Autodesk Fusion 360 part; units mm, degrees
(part 7 of 8)
  spline S13 degree 5 poles (6.6784, -162.4797) (6.7115, -162.4181) (6.7775, -162.295) (6.8761, -162.1103) (7.0066, -161.8637) (7.1683, -161.555) (7.3285, -161.246) (7.4872, -160.9366) (7.6444, -160.6268) (7.8, -160.3167) (7.9541, -160.0061) (8.1066, -159.6952) (8.2576, -159.3839) (8.407, -159.0722) (8.5549, -158.7602) (8.7011, -158.4478) (8.8457, -158.1351) (8.9887, -157.822) (9.1301, -157.5085) (9.2698, -157.1947) (9.4079, -156.8806) (9.5443, -156.5661) (9.679, -156.2513) (9.812, -155.9362) (9.9433, -155.6207) (10.0728, -155.3049) (10.2006, -154.9888) (10.3267, -154.6723) (10.4509, -154.3556) (10.5734, -154.0385) (10.694, -153.7211) (10.8129, -153.4035) (10.9298, -153.0855) (11.0449, -152.7672) (11.158, -152.4487) (11.2693, -152.1299) (11.3786, -151.8107) (11.486, -151.4913) (11.5914, -151.1717) (11.6948, -150.8517) (11.7962, -150.5315) (11.8955, -150.2111) (11.9926, -149.8904) (12.0876, -149.5694) (12.1804, -149.2482) (12.271, -148.9268) (12.3594, -148.6051) (12.4457, -148.2833) (12.5297, -147.9611) (12.6115, -147.6388) (12.6907, -147.3163) (12.7674, -146.9936) (12.8414, -146.6706) (12.9127, -146.3475) (12.9813, -146.0243) (13.0473, -145.7008) (13.1109, -145.3772) (13.1722, -145.0534) (13.231, -144.7295) (13.2868, -144.4055) (13.3392, -144.0813) (13.3875, -143.757) (13.4313, -143.4326) (13.4707, -143.1082) (13.5063, -142.7837) (13.539, -142.4591) (13.5696, -142.1346) (13.598, -141.81) (13.6235, -141.4854) (13.6434, -141.161) (13.6541, -140.8368) (13.6525, -140.5776) (13.6443, -140.3834) (13.6355, -140.254) (13.6303, -140.1893) knots -1 -1 -1 -1 -1 -1 -0.98571429 -0.97142857 -0.95714286 -0.94285714 -0.92857143 -0.91428571 -0.9 -0.88571429 -0.87142857 -0.85714286 -0.84285714 -0.82857143 -0.81428571 -0.8 -0.78571429 -0.77142857 -0.75714286 -0.74285714 -0.72857143 -0.71428571 -0.7 -0.68571429 -0.67142857 -0.65714286 -0.64285714 -0.62857143 -0.61428571 -0.6 -0.58571429 -0.57142857 -0.55714286 -0.54285714 -0.52857143 -0.51428571 -0.5 -0.48571429 -0.47142857 -0.45714286 -0.44285714 -0.42857143 -0.41428571 -0.4 -0.38571429 -0.37142857 -0.35714286 -0.34285714 -0.32857143 -0.31428571 -0.3 -0.28571429 -0.27142857 -0.25714286 -0.24285714 -0.22857143 -0.21428571 -0.2 -0.18571429 -0.17142857 -0.15714286 -0.14285714 -0.12857143 -0.11428571 -0.1 -0.08571429 -0.07142857 -0.05714286 -0.04285714 -0.02857143 -0.01428571 0 0 0 0 0 0
  line L13 (13.6303, -140.1893) -> (13.2679, -135.6821)
  arc A27 (14.7048, -133.974) -> (13.2679, -135.6821) centre (14.8503, -135.5548) ccw
  arc A28 (14.7048, -133.974) -> (25.331, -132.5751) centre (2.1352, 2.5578) ccw
  arc A29 (27.1609, -133.853) -> (25.331, -132.5751) centre (25.5995, -134.1397) ccw
  line L14 (27.1609, -133.853) -> (27.9775, -138.3004)
  spline S14 degree 5 poles (27.9775, -138.3004) (27.9892, -138.3643) (28.0142, -138.4915) (28.0566, -138.6813) (28.1221, -138.9321) (28.2164, -139.2425) (28.3195, -139.5507) (28.4281, -139.8576) (28.5397, -140.1637) (28.6532, -140.4693) (28.7687, -140.7744) (28.8871, -141.0786) (29.0091, -141.3818) (29.1355, -141.6837) (29.266, -141.9845) (29.4005, -142.284) (29.5383, -142.5826) (29.6789, -142.8803) (29.8219, -143.1771) (29.9671, -143.4733) (30.1146, -143.7686) (30.2646, -144.0631) (30.417, -144.3568) (30.5721, -144.6495) (30.7297, -144.9414) (30.8897, -145.2324) (31.0521, -145.5226) (31.2166, -145.812) (31.3832, -146.1006) (31.5519, -146.3884) (31.7227, -146.6754) (31.8954, -146.9617) (32.0702, -147.2471) (32.2471, -147.5317) (32.4259, -147.8156) (32.6067, -148.0986) (32.7893, -148.3809) (32.9739, -148.6624) (33.1603, -148.9431) (33.3485, -149.2231) (33.5385, -149.5023) (33.7302, -149.7807) (33.9238, -150.0583) (34.119, -150.3352) (34.316, -150.6113) (34.5147, -150.8866) (34.7151, -151.1611) (34.9171, -151.4349) (35.1207, -151.708) (35.326, -151.9803) (35.5329, -152.2518) (35.7413, -152.5225) (35.9514, -152.7925) (36.1629, -153.0617) (36.3761, -153.3302) (36.5907, -153.5979) (36.8069, -153.8648) (37.0246, -154.131) (37.2438, -154.3964) (37.4644, -154.6611) (37.6865, -154.925) (37.91, -155.1881) (38.135, -155.4505) (38.3614, -155.7121) (38.5893, -155.9729) (38.8185, -156.233) (39.0491, -156.4923) (39.2811, -156.7509) (39.5144, -157.0087) (39.7491, -157.2657) (39.9852, -157.522) (40.1751, -157.7264) (40.3182, -157.8793) (40.4138, -157.9811) (40.4617, -158.032) knots 0 0 0 0 0 0 0.01428571 0.02857143 0.04285714 0.05714286 0.07142857 0.08571429 0.1 0.11428571 0.12857143 0.14285714 0.15714286 0.17142857 0.18571429 0.2 0.21428571 0.22857143 0.24285714 0.25714286 0.27142857 0.28571429 0.3 0.31428571 0.32857143 0.34285714 0.35714286 0.37142857 0.38571429 0.4 0.41428571 0.42857143 0.44285714 0.45714286 0.47142857 0.48571429 0.5 0.51428571 0.52857143 0.54285714 0.55714286 0.57142857 0.58571429 0.6 0.61428571 0.62857143 0.64285714 0.65714286 0.67142857 0.68571429 0.7 0.71428571 0.72857143 0.74285714 0.75714286 0.77142857 0.78571429 0.8 0.81428571 0.82857143 0.84285714 0.85714286 0.87142857 0.88571429 0.9 0.91428571 0.92857143 0.94285714 0.95714286 0.97142857 0.98571429 1 1 1 1 1 1
  arc A30 (40.4617, -158.032) -> (49.2384, -155.6803) centre (2.1352, 2.5578) ccw
  spline S15 degree 5 poles (49.2384, -155.6803) (49.2545, -155.6123) (49.2864, -155.4763) (49.3338, -155.2723) (49.3961, -155.0003) (49.4724, -154.6604) (49.5471, -154.3204) (49.6203, -153.9805) (49.6919, -153.6406) (49.762, -153.3007) (49.8305, -152.9608) (49.8973, -152.621) (49.9626, -152.2813) (50.0263, -151.9416) (50.0883, -151.6019) (50.1487, -151.2623) (50.2074, -150.9228) (50.2645, -150.5834) (50.32, -150.244) (50.3737, -149.9047) (50.4258, -149.5656) (50.4761, -149.2265) (50.5247, -148.8876) (50.5716, -148.5487) (50.6168, -148.21) (50.6602, -147.8715) (50.7018, -147.533) (50.7417, -147.1948) (50.7797, -146.8566) (50.816, -146.5187) (50.8504, -146.1809) (50.8829, -145.8433) (50.9136, -145.5059) (50.9424, -145.1687) (50.9692, -144.8317) (50.9942, -144.4949) (51.0172, -144.1584) (51.0383, -143.8221) (51.0573, -143.486) (51.0744, -143.1502) (51.0894, -142.8147) (51.1024, -142.4795) (51.1132, -142.1446) (51.1219, -141.81) (51.1284, -141.4757) (51.1327, -141.1418) (51.1349, -140.8082) (51.1349, -140.4749) (51.1327, -140.142) (51.1282, -139.8095) (51.1213, -139.4775) (51.1119, -139.1459) (51.0998, -138.8148) (51.085, -138.4843) (51.0675, -138.1543) (51.0476, -137.8248) (51.0253, -137.4957) (51.0007, -137.1671) (50.9736, -136.839) (50.9437, -136.5116) (50.9104, -136.1849) (50.8731, -135.8592) (50.8315, -135.5345) (50.7856, -135.2109) (50.736, -134.8882) (50.6836, -134.5663) (50.6291, -134.2449) (50.5726, -133.924) (50.5132, -133.6039) (50.4484, -133.2854) (50.3749, -132.9694) (50.3062, -132.7195) (50.248, -132.534) (50.2061, -132.4113) (50.1843, -132.3501) knots -1 -1 -1 -1 -1 -1 -0.98571429 -0.97142857 -0.95714286 -0.94285714 -0.92857143 -0.91428571 -0.9 -0.88571429 -0.87142857 -0.85714286 -0.84285714 -0.82857143 -0.81428571 -0.8 -0.78571429 -0.77142857 -0.75714286 -0.74285714 -0.72857143 -0.71428571 -0.7 -0.68571429 -0.67142857 -0.65714286 -0.64285714 -0.62857143 -0.61428571 -0.6 -0.58571429 -0.57142857 -0.55714286 -0.54285714 -0.52857143 -0.51428571 -0.5 -0.48571429 -0.47142857 -0.45714286 -0.44285714 -0.42857143 -0.41428571 -0.4 -0.38571429 -0.37142857 -0.35714286 -0.34285714 -0.32857143 -0.31428571 -0.3 -0.28571429 -0.27142857 -0.25714286 -0.24285714 -0.22857143 -0.21428571 -0.2 -0.18571429 -0.17142857 -0.15714286 -0.14285714 -0.12857143 -0.11428571 -0.1 -0.08571429 -0.07142857 -0.05714286 -0.04285714 -0.02857143 -0.01428571 0 0 0 0 0 0
  line L15 (50.1843, -132.3501) -> (48.6677, -128.0903)
  arc A31 (49.6135, -126.0686) -> (48.6677, -128.0903) centre (50.1633, -127.5578) ccw
  arc A32 (49.6135, -126.0686) -> (59.5156, -121.967) centre (2.1352, 2.5578) ccw
  arc A33 (61.6139, -122.7278) -> (59.5156, -121.967) centre (60.1799, -123.4088) ccw
  line L16 (61.6139, -122.7278) -> (63.5537, -126.8123)
  spline S16 degree 5 poles (63.5537, -126.8123) (63.5816, -126.871) (63.6387, -126.9874) (63.7287, -127.1598) (63.8569, -127.385) (64.0283, -127.6604) (64.2077, -127.9315) (64.392, -128.1998) (64.579, -128.4666) (64.7677, -128.7325) (64.9583, -128.9972) (65.1514, -129.2604) (65.3477, -129.5217) (65.5479, -129.7807) (65.7519, -130.0373) (65.9593, -130.2919) (66.1697, -130.5446) (66.3825, -130.7957) (66.5975, -131.0455) (66.8144, -131.294) (67.0333, -131.5411) (67.2544, -131.7867) (67.4776, -132.0309) (67.7032, -132.2736) (67.9309, -132.5147) (68.1608, -132.7544) (68.3928, -132.9927) (68.6266, -133.2296) (68.8623, -133.4652) (69.0997, -133.6996) (69.3389, -133.9326) (69.5799, -134.1644) (69.8226, -134.3949) (70.0671, -134.6241) (70.3133, -134.8519) (70.5611, -135.0786) (70.8107, -135.3039) (71.0618, -135.5281) (71.3145, -135.751) (71.5687, -135.9727) (71.8245, -136.1932) (72.0818, -136.4125) (72.3406, -136.6305) (72.6008, -136.8474) (72.8626, -137.0631) (73.1257, -137.2777) (73.3903, -137.491) (73.6563, -137.7032) (73.9237, -137.9142) (74.1924, -138.1241) (74.4625, -138.3328) (74.734, -138.5404) (75.0067, -138.7468) (75.2808, -138.9521) (75.5561, -139.1562) (75.8328, -139.3593) (76.1107, -139.5611) (76.3898, -139.7619) (76.6702, -139.9616) (76.9518, -140.1601) (77.2347, -140.3575) (77.5187, -140.5538) (77.8039, -140.749) (78.0903, -140.9431) (78.3779, -141.1361) (78.6666, -141.328) (78.9565, -141.5188) (79.2475, -141.7085) (79.5396, -141.8971) (79.8328, -142.0846) (80.1272, -142.2711) (80.3635, -142.4194) (80.5413, -142.5301) (80.66, -142.6037) (80.7195, -142.6404) knots 0 0 0 0 0 0 0.01428571 0.02857143 0.04285714 0.05714286 0.07142857 0.08571429 0.1 0.11428571 0.12857143 0.14285714 0.15714286 0.17142857 0.18571429 0.2 0.21428571 0.22857143 0.24285714 0.25714286 0.27142857 0.28571429 0.3 0.31428571 0.32857143 0.34285714 0.35714286 0.37142857 0.38571429 0.4 0.41428571 0.42857143 0.44285714 0.45714286 0.47142857 0.48571429 0.5 0.51428571 0.52857143 0.54285714 0.55714286 0.57142857 0.58571429 0.6 0.61428571 0.62857143 0.64285714 0.65714286 0.67142857 0.68571429 0.7 0.71428571 0.72857143 0.74285714 0.75714286 0.77142857 0.78571429 0.8 0.81428571 0.82857143 0.84285714 0.85714286 0.87142857 0.88571429 0.9 0.91428571 0.92857143 0.94285714 0.95714286 0.97142857 0.98571429 1 1 1 1 1 1
  arc A34 (80.7195, -142.6404) -> (88.5885, -138.0973) centre (2.1352, 2.5578) ccw
  spline S17 degree 5 poles (88.5885, -138.0973) (88.5864, -138.0274) (88.582, -137.8878) (88.575, -137.6785) (88.5647, -137.3997) (88.5504, -137.0515) (88.5347, -136.7038) (88.5174, -136.3565) (88.4986, -136.0097) (88.4783, -135.6632) (88.4565, -135.3172) (88.4331, -134.9717) (88.4082, -134.6266) (88.3818, -134.282) (88.3538, -133.9379) (88.3243, -133.5942) (88.2931, -133.2511) (88.2604, -132.9084) (88.2261, -132.5663) (88.1902, -132.2247) (88.1527, -131.8836) (88.1136, -131.543) (88.0729, -131.2031) (88.0305, -130.8636) (87.9864, -130.5248) (87.9407, -130.1865) (87.8933, -129.8488) (87.8443, -129.5118) (87.7935, -129.1753) (87.7411, -128.8395) (87.6869, -128.5043) (87.6309, -128.1698) (87.5732, -127.836) (87.5137, -127.5028) (87.4525, -127.1703) (87.3894, -126.8386) (87.3245, -126.5076) (87.2578, -126.1773) (87.1893, -125.8477) (87.1189, -125.519) (87.0465, -125.191) (86.9723, -124.8638) (86.896, -124.5375) (86.8178, -124.2121) (86.7376, -123.8875) (86.6553, -123.5638) (86.5711, -123.241) (86.4849, -122.9191) (86.3966, -122.5982) (86.3062, -122.2782) (86.2136, -121.9592) (86.1187, -121.6414) (86.0213, -121.3247) (85.9214, -121.0093) (85.8192, -120.695) (85.7147, -120.3819) (85.608, -120.0698) (85.4991, -119.7588) (85.3881, -119.4489) (85.2744, -119.1403) (85.1577, -118.8334) (85.0374, -118.5284) (84.9132, -118.2256) (84.7851, -117.9249) (84.6536, -117.6261) (84.5197, -117.3287) (84.3838, -117.0323) (84.2462, -116.737) (84.106, -116.4432) (83.961, -116.1523) (83.8082, -115.8661) (83.6772, -115.6425) (83.5729, -115.4784) (83.5006, -115.3707) (83.4638, -115.3172) knots -1 -1 -1 -1 -1 -1 -0.98571429 -0.97142857 -0.95714286 -0.94285714 -0.92857143 -0.91428571 -0.9 -0.88571429 -0.87142857 -0.85714286 -0.84285714 -0.82857143 -0.81428571 -0.8 -0.78571429 -0.77142857 -0.75714286 -0.74285714 -0.72857143 -0.71428571 -0.7 -0.68571429 -0.67142857 -0.65714286 -0.64285714 -0.62857143 -0.61428571 -0.6 -0.58571429 -0.57142857 -0.55714286 -0.54285714 -0.52857143 -0.51428571 -0.5 -0.48571429 -0.47142857 -0.45714286 -0.44285714 -0.42857143 -0.41428571 -0.4 -0.38571429 -0.37142857 -0.35714286 -0.34285714 -0.32857143 -0.31428571 -0.3 -0.28571429 -0.27142857 -0.25714286 -0.24285714 -0.22857143 -0.21428571 -0.2 -0.18571429 -0.17142857 -0.15714286 -0.14285714 -0.12857143 -0.11428571 -0.1 -0.08571429 -0.07142857 -0.05714286 -0.04285714 -0.02857143 -0.01428571 0 0 0 0 0 0
  line L17 (83.4638, -115.3172) -> (80.8964, -111.5951)
  arc A35 (81.2867, -109.3974) -> (80.8964, -111.5951) centre (82.2032, -110.6937) ccw
  arc A36 (81.2867, -109.3974) -> (89.7898, -102.8728) centre (2.1352, 2.5578) ccw
  arc A37 (92.0135, -103.0646) -> (89.7898, -102.8728) centre (90.8047, -104.0935) ccw
  line L18 (92.0135, -103.0646) -> (94.9444, -106.5079)
  spline S18 degree 5 poles (94.9444, -106.5079) (94.9865, -106.5573) (95.0718, -106.655) (95.2033, -106.7982) (95.3854, -106.9826) (95.6223, -107.2043) (95.8657, -107.4196) (96.1132, -107.6311) (96.3629, -107.8404) (96.614, -108.0484) (96.8666, -108.2547) (97.1212, -108.459) (97.3785, -108.6606) (97.6389, -108.8589) (97.9023, -109.0541) (98.1686, -109.2463) (98.4372, -109.4359) (98.7078, -109.6234) (98.9801, -109.809) (99.2539, -109.9929) (99.5293, -110.1749) (99.8064, -110.355) (100.0853, -110.5331) (100.3659, -110.7091) (100.6483, -110.8831) (100.9325, -111.0551) (101.2182, -111.2252) (101.5053, -111.3935) (101.794, -111.5601) (102.084, -111.725) (102.3753, -111.8883) (102.6681, -112.0498) (102.9622, -112.2096) (103.2576, -112.3676) (103.5544, -112.524) (103.8525, -112.6788) (104.1518, -112.8319) (104.4524, -112.9834) (104.7542, -113.1333) (105.0571, -113.2817) (105.3613, -113.4284) (105.6665, -113.5737) (105.973, -113.7173) (106.2805, -113.8595) (106.5891, -114.0001) (106.8989, -114.1392) (107.2097, -114.2768) (107.5215, -114.4129) (107.8344, -114.5475) (108.1483, -114.6807) (108.4632, -114.8124) (108.7791, -114.9426) (109.096, -115.0714) (109.4139, -115.1988) (109.7327, -115.3247) (110.0524, -115.4492) (110.3731, -115.5723) (110.6947, -115.694) (111.0172, -115.8143) (111.3406, -115.9331) (111.6649, -116.0506) (111.9901, -116.1667) (112.3161, -116.2815) (112.643, -116.3948) (112.9707, -116.5068) (113.2993, -116.6174) (113.6286, -116.7267) (113.9588, -116.8346) (114.2898, -116.9412) (114.6216, -117.0464) (114.9542, -117.1504) (115.2208, -117.2324) (115.4212, -117.2933) (115.5549, -117.3337) (115.6218, -117.3538) knots 0 0 0 0 0 0 0.01428571 0.02857143 0.04285714 0.05714286 0.07142857 0.08571429 0.1 0.11428571 0.12857143 0.14285714 0.15714286 0.17142857 0.18571429 0.2 0.21428571 0.22857143 0.24285714 0.25714286 0.27142857 0.28571429 0.3 0.31428571 0.32857143 0.34285714 0.35714286 0.37142857 0.38571429 0.4 0.41428571 0.42857143 0.44285714 0.45714286 0.47142857 0.48571429 0.5 0.51428571 0.52857143 0.54285714 0.55714286 0.57142857 0.58571429 0.6 0.61428571 0.62857143 0.64285714 0.65714286 0.67142857 0.68571429 0.7 0.71428571 0.72857143 0.74285714 0.75714286 0.77142857 0.78571429 0.8 0.81428571 0.82857143 0.84285714 0.85714286 0.87142857 0.88571429 0.9 0.91428571 0.92857143 0.94285714 0.95714286 0.97142857 0.98571429 1 1 1 1 1 1
  arc A38 (115.6218, -117.3538) -> (122.0469, -110.9288) centre (2.1352, 2.5578) ccw
  spline S19 degree 5 poles (122.0469, -110.9288) (122.0267, -110.8619) (121.9864, -110.7282) (121.9254, -110.5278) (121.8434, -110.2611) (121.7395, -109.9286) (121.6342, -109.5968) (121.5277, -109.2658) (121.4197, -108.9356) (121.3105, -108.6062) (121.1998, -108.2777) (121.0878, -107.95) (120.9745, -107.6231) (120.8598, -107.297) (120.7437, -106.9719) (120.6262, -106.6476) (120.5073, -106.3242) (120.387, -106.0017) (120.2653, -105.6801) (120.1423, -105.3594) (120.0177, -105.0396) (119.8918, -104.7208) (119.7645, -104.403) (119.6357, -104.0861) (119.5054, -103.7702) (119.3737, -103.4553) (119.2406, -103.1414) (119.1059, -102.8285) (118.9698, -102.5166) (118.8322, -102.2058) (118.6931, -101.8961) (118.5525, -101.5875) (118.4104, -101.2799) (118.2667, -100.9735) (118.1215, -100.6682) (117.9747, -100.3641) (117.8263, -100.0612) (117.6764, -99.7594) (117.5249, -99.4588) (117.3718, -99.1595) (117.2171, -98.8614) (117.0607, -98.5646) (116.9026, -98.2691) (116.7428, -97.975) (116.5813, -97.6823) (116.4181, -97.3909) (116.2532, -97.1009) (116.0866, -96.8123) (115.9182, -96.5251) (115.7481, -96.2394) (115.5761, -95.9553) (115.4021, -95.6729) (115.2261, -95.3922) (115.048, -95.1134) (114.8679, -94.8363) (114.6859, -94.5609) (114.5021, -94.287) (114.3164, -94.0148) (114.1289, -93.7442) (113.9393, -93.4756) (113.7471, -93.2093) (113.552, -92.9459) (113.3536, -92.6855) (113.1521, -92.4282) (112.9478, -92.1736) (112.7414, -91.921) (112.5335, -91.6699) (112.3241, -91.4202) (112.1126, -91.1727) (111.8973, -90.9293) (111.6756, -90.6924) (111.4912, -90.5103) (111.348, -90.3788) (111.2503, -90.2934) (111.2009, -90.2514) knots -1 -1 -1 -1 -1 -1 -0.98571429 -0.97142857 -0.95714286 -0.94285714 -0.92857143 -0.91428571 -0.9 -0.88571429 -0.87142857 -0.85714286 -0.84285714 -0.82857143 -0.81428571 -0.8 -0.78571429 -0.77142857 -0.75714286 -0.74285714 -0.72857143 -0.71428571 -0.7 -0.68571429 -0.67142857 -0.65714286 -0.64285714 -0.62857143 -0.61428571 -0.6 -0.58571429 -0.57142857 -0.55714286 -0.54285714 -0.52857143 -0.51428571 -0.5 -0.48571429 -0.47142857 -0.45714286 -0.44285714 -0.42857143 -0.41428571 -0.4 -0.38571429 -0.37142857 -0.35714286 -0.34285714 -0.32857143 -0.31428571 -0.3 -0.28571429 -0.27142857 -0.25714286 -0.24285714 -0.22857143 -0.21428571 -0.2 -0.18571429 -0.17142857 -0.15714286 -0.14285714 -0.12857143 -0.11428571 -0.1 -0.08571429 -0.07142857 -0.05714286 -0.04285714 -0.02857143 -0.01428571 0 0 0 0 0 0
  line L19 (111.2009, -90.2514) -> (107.7576, -87.3205)
  arc A39 (107.5658, -85.0967) -> (107.7576, -87.3205) centre (108.7866, -86.1116) ccw
  arc A40 (107.5658, -85.0967) -> (114.0905, -76.5937) centre (2.1352, 2.5578) ccw
  arc A41 (116.2881, -76.2033) -> (114.0905, -76.5937) centre (115.3867, -77.5101) ccw
  line L20 (116.2881, -76.2033) -> (120.0103, -78.7708)
  spline S20 degree 5 poles (120.0103, -78.7708) (120.0637, -78.8076) (120.1714, -78.8799) (120.3355, -78.9842) (120.5592, -79.1151) (120.8453, -79.268) (121.1362, -79.413) (121.43, -79.5532) (121.7253, -79.6908) (122.0217, -79.8266) (122.3191, -79.9606) (122.6179, -80.092) (122.9186, -80.2201) (123.2215, -80.3443) (123.5264, -80.4646) (123.8333, -80.5814) (124.1419, -80.695) (124.4518, -80.8061) (124.7628, -80.9149) (125.0749, -81.0216) (125.3881, -81.1262) (125.7023, -81.2284) (126.0178, -81.3283) (126.3344, -81.4256) (126.6522, -81.5206) (126.9712, -81.6132) (127.2912, -81.7036) (127.6122, -81.7919) (127.9341, -81.8781) (128.2569, -81.9623) (128.5805, -82.0446) (128.9051, -82.1248) (129.2305, -82.203) (129.5569, -82.2793) (129.884, -82.3535) (130.212, -82.4258) (130.5408, -82.4962) (130.8703, -82.5648) (131.2006, -82.6315) (131.5316, -82.6964) (131.8634, -82.7594) (132.1958, -82.8207) (132.529, -82.8802) (132.8628, -82.9379) (133.1974, -82.9938) (133.5325, -83.048) (133.8684, -83.1005) (134.2048, -83.1513) (134.5419, -83.2003) (134.8795, -83.2477) (135.2178, -83.2934) (135.5567, -83.3374) (135.8961, -83.3798) (136.2361, -83.4206) (136.5766, -83.4597) (136.9177, -83.4972) (137.2593, -83.5331) (137.6014, -83.5674) (137.9441, -83.6001) (138.2872, -83.6312) (138.6309, -83.6608) (138.975, -83.6888) (139.3196, -83.7152) (139.6647, -83.7401) (140.0103, -83.7634) (140.3563, -83.7853) (140.7027, -83.8056) (141.0496, -83.8244) (141.3969, -83.8416) (141.7446, -83.8574) (142.0927, -83.8717) (142.3715, -83.8819) (142.5808, -83.889) (142.7205, -83.8933) (142.7903, -83.8954) knots 0 0 0 0 0 0 0.01428571 0.02857143 0.04285714 0.05714286 0.07142857 0.08571429 0.1 0.11428571 0.12857143 0.14285714 0.15714286 0.17142857 0.18571429 0.2 0.21428571 0.22857143 0.24285714 0.25714286 0.27142857 0.28571429 0.3 0.31428571 0.32857143 0.34285714 0.35714286 0.37142857 0.38571429 0.4 0.41428571 0.42857143 0.44285714 0.45714286 0.47142857 0.48571429 0.5 0.51428571 0.52857143 0.54285714 0.55714286 0.57142857 0.58571429 0.6 0.61428571 0.62857143 0.64285714 0.65714286 0.67142857 0.68571429 0.7 0.71428571 0.72857143 0.74285714 0.75714286 0.77142857 0.78571429 0.8 0.81428571 0.82857143 0.84285714 0.85714286 0.87142857 0.88571429 0.9 0.91428571 0.92857143 0.94285714 0.95714286 0.97142857 0.98571429 1 1 1 1 1 1
  arc A42 (142.7903, -83.8954) -> (147.3335, -76.0264) centre (2.1352, 2.5578) ccw
  spline S21 degree 5 poles (147.3335, -76.0264) (147.2967, -75.967) (147.2231, -75.8483) (147.1124, -75.6705) (146.9641, -75.4342) (146.7777, -75.1398) (146.5902, -74.8466) (146.4015, -74.5545) (146.2118, -74.2635) (146.021, -73.9736) (145.8291, -73.6849) (145.6361, -73.3973) (145.442, -73.1109) (145.2468, -72.8257) (145.0505, -72.5416) (144.8531, -72.2588) (144.6546, -71.9772) (144.4549, -71.6968) (144.2542, -71.4176) (144.0523, -71.1397) (143.8493, -70.8631) (143.6451, -70.5877) (143.4398, -70.3137) (143.2334, -70.0409) (143.0258, -69.7695) (142.8171, -69.4994) (142.6073, -69.2307) (142.3962, -68.9633) (142.1841, -68.6973) (141.9707, -68.4327) (141.7562, -68.1695) (141.5405, -67.9078) (141.3236, -67.6475) (141.1055, -67.3887) (140.8862, -67.1315) (140.6657, -66.8757) (140.444, -66.6214) (140.2211, -66.3687) (139.997, -66.1176) (139.7716, -65.8681) (139.545, -65.6202) (139.3171, -65.374) (139.0879, -65.1296) (138.8574, -64.8868) (138.6257, -64.6459) (138.3926, -64.4067) (138.1583, -64.1692) (137.9227, -63.9336) (137.6857, -63.6998) (137.4474, -63.4678) (137.2078, -63.2379) (136.9666, -63.0101) (136.7239, -62.7846) (136.4798, -62.5613) (136.2341, -62.3403) (135.987, -62.1214) (135.7385, -61.9045) (135.4888, -61.6895) (135.2376, -61.4767) (134.9849, -61.2663) (134.7304, -61.0588) (134.4737, -60.8549) (134.2147, -60.6547) (133.9534, -60.4584) (133.6902, -60.2653) (133.4255, -60.0747) (133.1597, -59.886) (132.8928, -59.699) (132.6245, -59.5147) (132.3535, -59.3353) (132.078, -59.1639) (131.8528, -59.0357) (131.6805, -58.9457) (131.564, -58.8885) (131.5054, -58.8607) knots -1 -1 -1 -1 -1 -1 -0.98571429 -0.97142857 -0.95714286 -0.94285714 -0.92857143 -0.91428571 -0.9 -0.88571429 -0.87142857 -0.85714286 -0.84285714 -0.82857143 -0.81428571 -0.8 -0.78571429 -0.77142857 -0.75714286 -0.74285714 -0.72857143 -0.71428571 -0.7 -0.68571429 -0.67142857 -0.65714286 -0.64285714 -0.62857143 -0.61428571 -0.6 -0.58571429 -0.57142857 -0.55714286 -0.54285714 -0.52857143 -0.51428571 -0.5 -0.48571429 -0.47142857 -0.45714286 -0.44285714 -0.42857143 -0.41428571 -0.4 -0.38571429 -0.37142857 -0.35714286 -0.34285714 -0.32857143 -0.31428571 -0.3 -0.28571429 -0.27142857 -0.25714286 -0.24285714 -0.22857143 -0.21428571 -0.2 -0.18571429 -0.17142857 -0.15714286 -0.14285714 -0.12857143 -0.11428571 -0.1 -0.08571429 -0.07142857 -0.05714286 -0.04285714 -0.02857143 -0.01428571 0 0 0 0 0 0
  line L21 (131.5054, -58.8607) -> (127.4208, -56.9209)
  arc A43 (126.66, -54.8225) -> (127.4208, -56.9209) centre (128.1018, -55.4869) ccw
  arc A44 (126.66, -54.8225) -> (130.7616, -44.9205) centre (2.1352, 2.5578) ccw
  arc A45 (132.7833, -43.9747) -> (130.7616, -44.9205) centre (132.2509, -45.4702) ccw
  line L22 (132.7833, -43.9747) -> (137.0432, -45.4913)
  spline S22 degree 5 poles (137.0432, -45.4913) (137.1043, -45.513) (137.2271, -45.555) (137.4125, -45.6132) (137.6625, -45.6818) (137.9784, -45.7554) (138.2969, -45.8202) (138.617, -45.8796) (138.9379, -45.936) (139.2593, -45.9906) (139.5813, -46.043) (139.9039, -46.0926) (140.2275, -46.1385) (140.5522, -46.1801) (140.8779, -46.2174) (141.2046, -46.2507) (141.5321, -46.2806) (141.8601, -46.3077) (142.1887, -46.3323) (142.5178, -46.3546) (142.8473, -46.3745) (143.1773, -46.3919) (143.5079, -46.4067) (143.8389, -46.4189) (144.1705, -46.4283) (144.5026, -46.4352) (144.8351, -46.4397) (145.1679, -46.4419) (145.5012, -46.4419) (145.8348, -46.4397) (146.1687, -46.4353) (146.503, -46.4288) (146.8376, -46.4202) (147.1725, -46.4094) (147.5077, -46.3964) (147.8433, -46.3814) (148.1791, -46.3643) (148.5151, -46.3452) (148.8514, -46.3242) (149.188, -46.3012) (149.5247, -46.2762) (149.8617, -46.2493) (150.1989, -46.2206) (150.5363, -46.1899) (150.8739, -46.1573) (151.2117, -46.1229) (151.5497, -46.0867) (151.8878, -46.0487) (152.2261, -46.0088) (152.5645, -45.9672) (152.9031, -45.9238) (153.2418, -45.8786) (153.5806, -45.8317) (153.9195, -45.7831) (154.2586, -45.7327) (154.5978, -45.6807) (154.937, -45.6269) (155.2764, -45.5715) (155.6158, -45.5144) (155.9553, -45.4557) (156.2949, -45.3953) (156.6346, -45.3332) (156.9743, -45.2696) (157.3141, -45.2043) (157.6539, -45.1374) (157.9937, -45.069) (158.3336, -44.9989) (158.6735, -44.9273) (159.0134, -44.8541) (159.3534, -44.7793) (159.6934, -44.703) (159.9653, -44.6408) (160.1693, -44.5934) (160.3053, -44.5614) (160.3733, -44.5454) knots 0 0 0 0 0 0 0.01428571 0.02857143 0.04285714 0.05714286 0.07142857 0.08571429 0.1 0.11428571 0.12857143 0.14285714 0.15714286 0.17142857 0.18571429 0.2 0.21428571 0.22857143 0.24285714 0.25714286 0.27142857 0.28571429 0.3 0.31428571 0.32857143 0.34285714 0.35714286 0.37142857 0.38571429 0.4 0.41428571 0.42857143 0.44285714 0.45714286 0.47142857 0.48571429 0.5 0.51428571 0.52857143 0.54285714 0.55714286 0.57142857 0.58571429 0.6 0.61428571 0.62857143 0.64285714 0.65714286 0.67142857 0.68571429 0.7 0.71428571 0.72857143 0.74285714 0.75714286 0.77142857 0.78571429 0.8 0.81428571 0.82857143 0.84285714 0.85714286 0.87142857 0.88571429 0.9 0.91428571 0.92857143 0.94285714 0.95714286 0.97142857 0.98571429 1 1 1 1 1 1
  arc A46 (160.3733, -44.5454) -> (162.725, -35.7687) centre (2.1352, 2.5578) ccw
  spline S23 degree 5 poles (162.725, -35.7687) (162.6742, -35.7208) (162.5724, -35.6252) (162.4194, -35.4821) (162.215, -35.2922) (161.9587, -35.0561) (161.7017, -34.8214) (161.4439, -34.5881) (161.1853, -34.3561) (160.926, -34.1255) (160.6659, -33.8962) (160.4051, -33.6684) (160.1435, -33.442) (159.8811, -33.217) (159.618, -32.9935) (159.3541, -32.7714) (159.0894, -32.5507) (158.824, -32.3316) (158.5578, -32.1139) (158.2909, -31.8977) (158.0232, -31.6831) (157.7547, -31.4699) (157.4855, -31.2583) (157.2155, -31.0483) (156.9448, -30.8398) (156.6733, -30.633) (156.401, -30.4277) (156.128, -30.224) (155.8542, -30.022) (155.5796, -29.8217) (155.3043, -29.623) (155.0282, -29.426) (154.7513, -29.2307) (154.4737, -29.0372) (154.1953, -28.8455) (153.9161, -28.6555) (153.6362, -28.4673) (153.3554, -28.2809) (153.0739, -28.0963) (152.7917, -27.9136) (152.5086, -27.7329) (152.2248, -27.554) (151.9401, -27.3772) (151.6547, -27.2024) (151.3685, -27.0296) (151.0814, -26.8589) (150.7936, -26.6902) (150.505, -26.5236) (150.2157, -26.359) (149.9255, -26.1967) (149.6345, -26.0366) (149.3426, -25.879) (149.0498, -25.724) (148.7562, -25.5715) (148.4616, -25.4216) (148.1663, -25.2741) (147.8702, -25.1289) (147.5733, -24.9859) (147.2756, -24.8453) (146.9771, -24.7075) (146.6775, -24.573) (146.3768, -24.4424) (146.0748, -24.3161) (145.7716, -24.1941) (145.4674, -24.0757) (145.1624, -23.9601) (144.8567, -23.8466) (144.5506, -23.7351) (144.2437, -23.6265) (143.9355, -23.5233) (143.6251, -23.4291) (143.3743, -23.3635) (143.1846, -23.3212) (143.0573, -23.2962) (142.9935, -23.2845) knots -1 -1 -1 -1 -1 -1 -0.98571429 -0.97142857 -0.95714286 -0.94285714 -0.92857143 -0.91428571 -0.9 -0.88571429 -0.87142857 -0.85714286 -0.84285714 -0.82857143 -0.81428571 -0.8 -0.78571429 -0.77142857 -0.75714286 -0.74285714 -0.72857143 -0.71428571 -0.7 -0.68571429 -0.67142857 -0.65714286 -0.64285714 -0.62857143 -0.61428571 -0.6 -0.58571429 -0.57142857 -0.55714286 -0.54285714 -0.52857143 -0.51428571 -0.5 -0.48571429 -0.47142857 -0.45714286 -0.44285714 -0.42857143 -0.41428571 -0.4 -0.38571429 -0.37142857 -0.35714286 -0.34285714 -0.32857143 -0.31428571 -0.3 -0.28571429 -0.27142857 -0.25714286 -0.24285714 -0.22857143 -0.21428571 -0.2 -0.18571429 -0.17142857 -0.15714286 -0.14285714 -0.12857143 -0.11428571 -0.1 -0.08571429 -0.07142857 -0.05714286 -0.04285714 -0.02857143 -0.01428571 0 0 0 0 0 0
  line L23 (142.9935, -23.2845) -> (138.546, -22.4679)
  arc A47 (137.2681, -20.6379) -> (138.546, -22.4679) centre (138.8327, -20.9065) ccw
  arc A48 (137.2681, -20.6379) -> (138.667, -10.0118) centre (2.1352, 2.5578) ccw
  arc A49 (140.3751, -8.5749) -> (138.667, -10.0118) centre (140.2479, -10.1573) ccw
  line L24 (140.3751, -8.5749) -> (144.8823, -8.9373)
  spline S24 degree 5 poles (144.8823, -8.9373) (144.947, -8.9425) (145.0764, -8.9512) (145.2707, -8.9595) (145.5298, -8.9611) (145.8541, -8.9504) (146.1785, -8.9305) (146.503, -8.905) (146.8276, -8.8765) (147.1522, -8.846) (147.4767, -8.8133) (147.8012, -8.7777) (148.1257, -8.7383) (148.45, -8.6944) (148.7743, -8.6461) (149.0985, -8.5938) (149.4225, -8.5379) (149.7464, -8.4792) (150.0702, -8.4179) (150.3938, -8.3543) (150.7173, -8.2882) (151.0406, -8.2196) (151.3637, -8.1484) (151.6866, -8.0744) (152.0093, -7.9977) (152.3319, -7.9184) (152.6542, -7.8367) (152.9763, -7.7527) (153.2982, -7.6664) (153.6198, -7.5779) (153.9413, -7.4873) (154.2625, -7.3945) (154.5834, -7.2996) (154.9041, -7.2024) (155.2246, -7.1032) (155.5448, -7.0018) (155.8647, -6.8984) (156.1844, -6.793) (156.5038, -6.6856) (156.8229, -6.5763) (157.1417, -6.465) (157.4603, -6.3518) (157.7785, -6.2368) (158.0965, -6.1198) (158.4142, -6.001) (158.7315, -5.8804) (159.0486, -5.7579) (159.3654, -5.6336) (159.6818, -5.5076) (159.9979, -5.3798) (160.3137, -5.2502) (160.6292, -5.1189) (160.9443, -4.9859) (161.2592, -4.8512) (161.5736, -4.7148) (161.8878, -4.5768) (162.2016, -4.4371) (162.515, -4.2957) (162.8281, -4.1527) (163.1408, -4.0081) (163.4532, -3.8618) (163.7653, -3.714) (164.0769, -3.5646) (164.3882, -3.4136) (164.6991, -3.2611) (165.0097, -3.107) (165.3199, -2.9513) (165.6296, -2.7942) (165.9391, -2.6355) (166.2481, -2.4753) (166.5567, -2.3136) (166.8033, -2.1831) (166.9881, -2.0845) (167.1112, -2.0185) (167.1727, -1.9854) knots 0 0 0 0 0 0 0.01428571 0.02857143 0.04285714 0.05714286 0.07142857 0.08571429 0.1 0.11428571 0.12857143 0.14285714 0.15714286 0.17142857 0.18571429 0.2 0.21428571 0.22857143 0.24285714 0.25714286 0.27142857 0.28571429 0.3 0.31428571 0.32857143 0.34285714 0.35714286 0.37142857 0.38571429 0.4 0.41428571 0.42857143 0.44285714 0.45714286 0.47142857 0.48571429 0.5 0.51428571 0.52857143 0.54285714 0.55714286 0.57142857 0.58571429 0.6 0.61428571 0.62857143 0.64285714 0.65714286 0.67142857 0.68571429 0.7 0.71428571 0.72857143 0.74285714 0.75714286 0.77142857 0.78571429 0.8 0.81428571 0.82857143 0.84285714 0.85714286 0.87142857 0.88571429 0.9 0.91428571 0.92857143 0.94285714 0.95714286 0.97142857 0.98571429 1 1 1 1 1 1
  arc A50 (167.1727, -1.9854) -> (167.1727, 7.101) centre (2.1352, 2.5578) ccw
  spline S25 degree 5 poles (167.1727, 7.101) (167.1112, 7.1341) (166.9881, 7.2001) (166.8033, 7.2987) (166.5567, 7.4292) (166.2481, 7.5909) (165.9391, 7.7511) (165.6296, 7.9098) (165.3199, 8.0669) (165.0097, 8.2226) (164.6991, 8.3767) (164.3882, 8.5292) (164.0769, 8.6802) (163.7653, 8.8296) (163.4532, 8.9774) (163.1408, 9.1237) (162.8281, 9.2683) (162.515, 9.4113) (162.2016, 9.5527) (161.8878, 9.6924) (161.5736, 9.8305) (161.2592, 9.9668) (160.9443, 10.1015) (160.6292, 10.2345) (160.3137, 10.3658) (159.9979, 10.4954) (159.6818, 10.6232) (159.3654, 10.7492) (159.0486, 10.8735) (158.7315, 10.996) (158.4142, 11.1166) (158.0965, 11.2354) (157.7785, 11.3524) (157.4603, 11.4675) (157.1417, 11.5806) (156.8229, 11.6919) (156.5038, 11.8012) (156.1844, 11.9086) (155.8647, 12.014) (155.5448, 12.1174) (155.2246, 12.2188) (154.9041, 12.318) (154.5834, 12.4152) (154.2625, 12.5101) (153.9413, 12.6029) (153.6198, 12.6936) (153.2982, 12.782) (152.9763, 12.8683) (152.6542, 12.9523) (152.3319, 13.034) (152.0093, 13.1133) (151.6866, 13.19) (151.3637, 13.264) (151.0406, 13.3352) (150.7173, 13.4038) (150.3938, 13.4699) (150.0702, 13.5335) (149.7464, 13.5948) (149.4225, 13.6535) (149.0985, 13.7094) (148.7743, 13.7617) (148.45, 13.81) (148.1257, 13.8539) (147.8012, 13.8933) (147.4767, 13.9289) (147.1522, 13.9616) (146.8276, 13.9921) (146.503, 14.0206) (146.1785, 14.0461) (145.8541, 14.066) (145.5298, 14.0767) (145.2707, 14.0751) (145.0764, 14.0668) (144.947, 14.0581) (144.8823, 14.0529) knots -1 -1 -1 -1 -1 -1 -0.98571429 -0.97142857 -0.95714286 -0.94285714 -0.92857143 -0.91428571 -0.9 -0.88571429 -0.87142857 -0.85714286 -0.84285714 -0.82857143 -0.81428571 -0.8 -0.78571429 -0.77142857 -0.75714286 -0.74285714 -0.72857143 -0.71428571 -0.7 -0.68571429 -0.67142857 -0.65714286 -0.64285714 -0.62857143 -0.61428571 -0.6 -0.58571429 -0.57142857 -0.55714286 -0.54285714 -0.52857143 -0.51428571 -0.5 -0.48571429 -0.47142857 -0.45714286 -0.44285714 -0.42857143 -0.41428571 -0.4 -0.38571429 -0.37142857 -0.35714286 -0.34285714 -0.32857143 -0.31428571 -0.3 -0.28571429 -0.27142857 -0.25714286 -0.24285714 -0.22857143 -0.21428571 -0.2 -0.18571429 -0.17142857 -0.15714286 -0.14285714 -0.12857143 -0.11428571 -0.1 -0.08571429 -0.07142857 -0.05714286 -0.04285714 -0.02857143 -0.01428571 0 0 0 0 0 0
  line L25 (144.8823, 14.0529) -> (140.3751, 13.6905)
  arc A51 (138.667, 15.1274) -> (140.3751, 13.6905) centre (140.2479, 15.2729) ccw
  arc A52 (138.667, 15.1274) -> (137.2681, 25.7536) centre (2.1352, 2.5578) ccw
  arc A53 (138.546, 27.5835) -> (137.2681, 25.7536) centre (138.8327, 26.0221) ccw
  line L26 (138.546, 27.5835) -> (142.9935, 28.4001)
  spline S26 degree 5 poles (142.9935, 28.4001) (143.0573, 28.4118) (143.1846, 28.4368) (143.3743, 28.4792) (143.6251, 28.5447) (143.9355, 28.6389) (144.2437, 28.7421) (144.5506, 28.8507) (144.8567, 28.9622) (145.1624, 29.0757) (145.4674, 29.1913) (145.7716, 29.3097) (146.0748, 29.4317) (146.3768, 29.558) (146.6775, 29.6886) (146.9771, 29.8231) (147.2756, 29.9609) (147.5733, 30.1015) (147.8702, 30.2445) (148.1663, 30.3897) (148.4616, 30.5372) (148.7562, 30.6871) (149.0498, 30.8396) (149.3426, 30.9946) (149.6345, 31.1522) (149.9255, 31.3123) (150.2157, 31.4746) (150.505, 31.6392) (150.7936, 31.8058) (151.0814, 31.9745) (151.3685, 32.1452) (151.6547, 32.318) (151.9401, 32.4928) (152.2248, 32.6696) (152.5086, 32.8485) (152.7917, 33.0292) (153.0739, 33.2119) (153.3554, 33.3965) (153.6362, 33.5829) (153.9161, 33.7711) (154.1953, 33.9611) (154.4737, 34.1528) (154.7513, 34.3463) (155.0282, 34.5416) (155.3043, 34.7386) (155.5796, 34.9373) (155.8542, 35.1376) (156.128, 35.3396) (156.401, 35.5433) (156.6733, 35.7486) (156.9448, 35.9554) (157.2155, 36.1639) (157.4855, 36.3739) (157.7547, 36.5855) (158.0232, 36.7987) (158.2909, 37.0133) (158.5578, 37.2295) (158.824, 37.4472) (159.0894, 37.6663) (159.3541, 37.887) (159.618, 38.1091) (159.8811, 38.3326) (160.1435, 38.5576) (160.4051, 38.784) (160.6659, 39.0118) (160.926, 39.2411) (161.1853, 39.4717) (161.4439, 39.7037) (161.7017, 39.937) (161.9587, 40.1717) (162.215, 40.4078) (162.4194, 40.5977) (162.5724, 40.7408) (162.6742, 40.8364) (162.725, 40.8843) knots 0 0 0 0 0 0 0.01428571 0.02857143 0.04285714 0.05714286 0.07142857 0.08571429 0.1 0.11428571 0.12857143 0.14285714 0.15714286 0.17142857 0.18571429 0.2 0.21428571 0.22857143 0.24285714 0.25714286 0.27142857 0.28571429 0.3 0.31428571 0.32857143 0.34285714 0.35714286 0.37142857 0.38571429 0.4 0.41428571 0.42857143 0.44285714 0.45714286 0.47142857 0.48571429 0.5 0.51428571 0.52857143 0.54285714 0.55714286 0.57142857 0.58571429 0.6 0.61428571 0.62857143 0.64285714 0.65714286 0.67142857 0.68571429 0.7 0.71428571 0.72857143 0.74285714 0.75714286 0.77142857 0.78571429 0.8 0.81428571 0.82857143 0.84285714 0.85714286 0.87142857 0.88571429 0.9 0.91428571 0.92857143 0.94285714 0.95714286 0.97142857 0.98571429 1 1 1 1 1 1
  arc A54 (162.725, 40.8843) -> (160.3733, 49.661) centre (2.1352, 2.5578) ccw
  spline S27 degree 5 poles (160.3733, 49.661) (160.3053, 49.677) (160.1693, 49.709) (159.9653, 49.7564) (159.6934, 49.8186) (159.3534, 49.8949) (159.0134, 49.9697) (158.6735, 50.0429) (158.3336, 50.1145) (157.9937, 50.1846) (157.6539, 50.253) (157.3141, 50.3199) (156.9743, 50.3852) (156.6346, 50.4488) (156.2949, 50.5109) (155.9553, 50.5713) (155.6158, 50.63) (155.2764, 50.6871) (154.937, 50.7425) (154.5978, 50.7963) (154.2586, 50.8483) (153.9195, 50.8987) (153.5806, 50.9473) (153.2418, 50.9942) (152.9031, 51.0394) (152.5645, 51.0828) (152.2261, 51.1244) (151.8878, 51.1643) (151.5497, 51.2023) (151.2117, 51.2386) (150.8739, 51.273) (150.5363, 51.3055) (150.1989, 51.3362) (149.8617, 51.3649) (149.5247, 51.3918) (149.188, 51.4168) (148.8514, 51.4398) (148.5151, 51.4608) (148.1791, 51.4799) (147.8433, 51.497) (147.5077, 51.512) (147.1725, 51.525) (146.8376, 51.5358) (146.503, 51.5444) (146.1687, 51.5509) (145.8348, 51.5553) (145.5012, 51.5575) (145.1679, 51.5575) (144.8351, 51.5553) (144.5026, 51.5508) (144.1705, 51.5439) (143.8389, 51.5345) (143.5079, 51.5224) (143.1773, 51.5076) (142.8473, 51.4901) (142.5178, 51.4702) (142.1887, 51.4479) (141.8601, 51.4233) (141.5321, 51.3962) (141.2046, 51.3663) (140.8779, 51.333) (140.5522, 51.2957) (140.2275, 51.2541) (139.9039, 51.2082) (139.5813, 51.1586) (139.2593, 51.1062) (138.9379, 51.0517) (138.617, 50.9952) (138.2969, 50.9358) (137.9784, 50.871) (137.6625, 50.7974) (137.4125, 50.7288) (137.2271, 50.6706) (137.1043, 50.6286) (137.0432, 50.6069) knots -1 -1 -1 -1 -1 -1 -0.98571429 -0.97142857 -0.95714286 -0.94285714 -0.92857143 -0.91428571 -0.9 -0.88571429 -0.87142857 -0.85714286 -0.84285714 -0.82857143 -0.81428571 -0.8 -0.78571429 -0.77142857 -0.75714286 -0.74285714 -0.72857143 -0.71428571 -0.7 -0.68571429 -0.67142857 -0.65714286 -0.64285714 -0.62857143 -0.61428571 -0.6 -0.58571429 -0.57142857 -0.55714286 -0.54285714 -0.52857143 -0.51428571 -0.5 -0.48571429 -0.47142857 -0.45714286 -0.44285714 -0.42857143 -0.41428571 -0.4 -0.38571429 -0.37142857 -0.35714286 -0.34285714 -0.32857143 -0.31428571 -0.3 -0.28571429 -0.27142857 -0.25714286 -0.24285714 -0.22857143 -0.21428571 -0.2 -0.18571429 -0.17142857 -0.15714286 -0.14285714 -0.12857143 -0.11428571 -0.1 -0.08571429 -0.07142857 -0.05714286 -0.04285714 -0.02857143 -0.01428571 0 0 0 0 0 0
  line L27 (137.0432, 50.6069) -> (132.7833, 49.0903)
  arc A55 (130.7616, 50.0361) -> (132.7833, 49.0903) centre (132.2509, 50.5858) ccw
  arc A56 (130.7616, 50.0361) -> (126.66, 59.9381) centre (2.1352, 2.5578) ccw
  arc A57 (127.4208, 62.0365) -> (126.66, 59.9381) centre (128.1018, 60.6025) ccw
  line L28 (127.4208, 62.0365) -> (131.5054, 63.9763)
  spline S28 degree 5 poles (131.5054, 63.9763) (131.564, 64.0041) (131.6805, 64.0613) (131.8528, 64.1513) (132.078, 64.2795) (132.3535, 64.4509) (132.6245, 64.6303) (132.8928, 64.8146) (133.1597, 65.0016) (133.4255, 65.1903) (133.6902, 65.3809) (133.9534, 65.574) (134.2147, 65.7703) (134.4737, 65.9705) (134.7304, 66.1745) (134.9849, 66.3819) (135.2376, 66.5923) (135.4888, 66.8051) (135.7385, 67.0201) (135.987, 67.237) (136.2341, 67.4559) (136.4798, 67.6769) (136.7239, 67.9002) (136.9666, 68.1257) (137.2078, 68.3535) (137.4474, 68.5834) (137.6857, 68.8154) (137.9227, 69.0492) (138.1583, 69.2849) (138.3926, 69.5223) (138.6257, 69.7615) (138.8574, 70.0024) (139.0879, 70.2452) (139.3171, 70.4896) (139.545, 70.7358) (139.7716, 70.9837) (139.997, 71.2332) (140.2211, 71.4844) (140.444, 71.737) (140.6657, 71.9913) (140.8862, 72.2471) (141.1055, 72.5043) (141.3236, 72.7631) (141.5405, 73.0234) (141.7562, 73.2851) (141.9707, 73.5483) (142.1841, 73.8129) (142.3962, 74.0789) (142.6073, 74.3463) (142.8171, 74.615) (143.0258, 74.8851) (143.2334, 75.1565) (143.4398, 75.4293) (143.6451, 75.7034) (143.8493, 75.9787) (144.0523, 76.2553) (144.2542, 76.5332) (144.4549, 76.8124) (144.6546, 77.0928) (144.8531, 77.3744) (145.0505, 77.6572) (145.2468, 77.9413) (145.442, 78.2265) (145.6361, 78.5129) (145.8291, 78.8005) (146.021, 79.0892) (146.2118, 79.3791) (146.4015, 79.6701) (146.5902, 79.9622) (146.7777, 80.2554) (146.9641, 80.5498) (147.1124, 80.7861) (147.2231, 80.9639) (147.2967, 81.0826) (147.3335, 81.142) knots 0 0 0 0 0 0 0.01428571 0.02857143 0.04285714 0.05714286 0.07142857 0.08571429 0.1 0.11428571 0.12857143 0.14285714 0.15714286 0.17142857 0.18571429 0.2 0.21428571 0.22857143 0.24285714 0.25714286 0.27142857 0.28571429 0.3 0.31428571 0.32857143 0.34285714 0.35714286 0.37142857 0.38571429 0.4 0.41428571 0.42857143 0.44285714 0.45714286 0.47142857 0.48571429 0.5 0.51428571 0.52857143 0.54285714 0.55714286 0.57142857 0.58571429 0.6 0.61428571 0.62857143 0.64285714 0.65714286 0.67142857 0.68571429 0.7 0.71428571 0.72857143 0.74285714 0.75714286 0.77142857 0.78571429 0.8 0.81428571 0.82857143 0.84285714 0.85714286 0.87142857 0.88571429 0.9 0.91428571 0.92857143 0.94285714 0.95714286 0.97142857 0.98571429 1 1 1 1 1 1
  arc A58 (147.3335, 81.142) -> (142.7903, 89.011) centre (2.1352, 2.5578) ccw
  spline S29 degree 5 poles (142.7903, 89.011) (142.7205, 89.0089) (142.5808, 89.0046) (142.3715, 88.9976) (142.0927, 88.9873) (141.7446, 88.973) (141.3969, 88.9572) (141.0496, 88.94) (140.7027, 88.9212) (140.3563, 88.9009) (140.0103, 88.879) (139.6647, 88.8557) (139.3196, 88.8308) (138.975, 88.8044) (138.6309, 88.7764) (138.2872, 88.7468) (137.9441, 88.7157) (137.6014, 88.683) (137.2593, 88.6487) (136.9177, 88.6128) (136.5766, 88.5753) (136.2361, 88.5362) (135.8961, 88.4954) (135.5567, 88.453) (135.2178, 88.409) (134.8795, 88.3633) (134.5419, 88.3159) (134.2048, 88.2669) (133.8684, 88.2161) (133.5325, 88.1636) (133.1974, 88.1094) (132.8628, 88.0535) (132.529, 87.9958) (132.1958, 87.9363) (131.8634, 87.875) (131.5316, 87.812) (131.2006, 87.7471) (130.8703, 87.6804) (130.5408, 87.6119) (130.212, 87.5414) (129.884, 87.4691) (129.5569, 87.3949) (129.2305, 87.3186) (128.9051, 87.2404) (128.5805, 87.1602) (128.2569, 87.0779) (127.9341, 86.9937) (127.6122, 86.9075) (127.2912, 86.8192) (126.9712, 86.7288) (126.6522, 86.6362) (126.3344, 86.5412) (126.0178, 86.4439) (125.7023, 86.344) (125.3881, 86.2418) (125.0749, 86.1372) (124.7628, 86.0305) (124.4518, 85.9217) (124.1419, 85.8106) (123.8333, 85.697) (123.5264, 85.5802) (123.2215, 85.4599) (122.9186, 85.3357) (122.6179, 85.2077) (122.3191, 85.0762) (122.0217, 84.9423) (121.7253, 84.8064) (121.43, 84.6688) (121.1362, 84.5286) (120.8453, 84.3836) (120.5592, 84.2308) (120.3355, 84.0998) (120.1714, 83.9955) (120.0637, 83.9232) (120.0103, 83.8864) knots -1 -1 -1 -1 -1 -1 -0.98571429 -0.97142857 -0.95714286 -0.94285714 -0.92857143 -0.91428571 -0.9 -0.88571429 -0.87142857 -0.85714286 -0.84285714 -0.82857143 -0.81428571 -0.8 -0.78571429 -0.77142857 -0.75714286 -0.74285714 -0.72857143 -0.71428571 -0.7 -0.68571429 -0.67142857 -0.65714286 -0.64285714 -0.62857143 -0.61428571 -0.6 -0.58571429 -0.57142857 -0.55714286 -0.54285714 -0.52857143 -0.51428571 -0.5 -0.48571429 -0.47142857 -0.45714286 -0.44285714 -0.42857143 -0.41428571 -0.4 -0.38571429 -0.37142857 -0.35714286 -0.34285714 -0.32857143 -0.31428571 -0.3 -0.28571429 -0.27142857 -0.25714286 -0.24285714 -0.22857143 -0.21428571 -0.2 -0.18571429 -0.17142857 -0.15714286 -0.14285714 -0.12857143 -0.11428571 -0.1 -0.08571429 -0.07142857 -0.05714286 -0.04285714 -0.02857143 -0.01428571 0 0 0 0 0 0
  line L29 (120.0103, 83.8864) -> (116.2881, 81.319)
  arc A59 (114.0905, 81.7093) -> (116.2881, 81.319) centre (115.3867, 82.6257) ccw
  arc A60 (114.0905, 81.7093) -> (107.5658, 90.2123) centre (2.1352, 2.5578) ccw
  arc A61 (107.7576, 92.4361) -> (107.5658, 90.2123) centre (108.7866, 91.2272) ccw
  line L30 (107.7576, 92.4361) -> (111.2009, 95.367)
  spline S30 degree 5 poles (111.2009, 95.367) (111.2503, 95.409) (111.348, 95.4944) (111.4912, 95.6259) (111.6756, 95.808) (111.8973, 96.0449) (112.1126, 96.2883) (112.3241, 96.5358) (112.5335, 96.7855) (112.7414, 97.0366) (112.9478, 97.2892) (113.1521, 97.5438) (113.3536, 97.8011) (113.552, 98.0615) (113.7471, 98.3249) (113.9393, 98.5912) (114.1289, 98.8598) (114.3164, 99.1304) (114.5021, 99.4026) (114.6859, 99.6765) (114.8679, 99.9519) (115.048, 100.229) (115.2261, 100.5078) (115.4021, 100.7885) (115.5761, 101.0709) (115.7481, 101.355) (115.9182, 101.6407) (116.0866, 101.9279) (116.2532, 102.2165) (116.4181, 102.5065) (116.5813, 102.7979) (116.7428, 103.0906) (116.9026, 103.3847) (117.0607, 103.6802) (117.2171, 103.977) (117.3718, 104.2751) (117.5249, 104.5744) (117.6764, 104.875) (117.8263, 105.1768) (117.9747, 105.4797) (118.1215, 105.7839) (118.2667, 106.0891) (118.4104, 106.3955) (118.5525, 106.7031) (118.6931, 107.0117) (118.8322, 107.3214) (118.9698, 107.6322) (119.1059, 107.9441) (119.2406, 108.257) (119.3737, 108.5709) (119.5054, 108.8858) (119.6357, 109.2017) (119.7645, 109.5186) (119.8918, 109.8364) (120.0177, 110.1552) (120.1423, 110.475) (120.2653, 110.7957) (120.387, 111.1173) (120.5073, 111.4398) (120.6262, 111.7632) (120.7437, 112.0875) (120.8598, 112.4127) (120.9745, 112.7387) (121.0878, 113.0656) (121.1998, 113.3933) (121.3105, 113.7218) (121.4197, 114.0512) (121.5277, 114.3814) (121.6342, 114.7124) (121.7395, 115.0442) (121.8434, 115.3767) (121.9254, 115.6434) (121.9864, 115.8438) (122.0267, 115.9775) (122.0469, 116.0444) knots 0 0 0 0 0 0 0.01428571 0.02857143 0.04285714 0.05714286 0.07142857 0.08571429 0.1 0.11428571 0.12857143 0.14285714 0.15714286 0.17142857 0.18571429 0.2 0.21428571 0.22857143 0.24285714 0.25714286 0.27142857 0.28571429 0.3 0.31428571 0.32857143 0.34285714 0.35714286 0.37142857 0.38571429 0.4 0.41428571 0.42857143 0.44285714 0.45714286 0.47142857 0.48571429 0.5 0.51428571 0.52857143 0.54285714 0.55714286 0.57142857 0.58571429 0.6 0.61428571 0.62857143 0.64285714 0.65714286 0.67142857 0.68571429 0.7 0.71428571 0.72857143 0.74285714 0.75714286 0.77142857 0.78571429 0.8 0.81428571 0.82857143 0.84285714 0.85714286 0.87142857 0.88571429 0.9 0.91428571 0.92857143 0.94285714 0.95714286 0.97142857 0.98571429 1 1 1 1 1 1
  arc A62 (122.0469, 116.0444) -> (115.6218, 122.4694) centre (2.1352, 2.5578) ccw
  spline S31 degree 5 poles (115.6218, 122.4694) (115.5549, 122.4493) (115.4212, 122.409) (115.2208, 122.348) (114.9542, 122.266) (114.6216, 122.1621) (114.2898, 122.0568) (113.9588, 121.9502) (113.6286, 121.8423) (113.2993, 121.733) (112.9707, 121.6224) (112.643, 121.5104) (112.3161, 121.3971) (111.9901, 121.2823) (111.6649, 121.1662) (111.3406, 121.0487) (111.0172, 120.9299) (110.6947, 120.8096) (110.3731, 120.6879) (110.0524, 120.5648) (109.7327, 120.4403) (109.4139, 120.3144) (109.096, 120.187) (108.7791, 120.0582) (108.4632, 119.928) (108.1483, 119.7963) (107.8344, 119.6631) (107.5215, 119.5285) (107.2097, 119.3924) (106.8989, 119.2548) (106.5891, 119.1157) (106.2805, 118.9751) (105.973, 118.833) (105.6665, 118.6893) (105.3613, 118.544) (105.0571, 118.3973) (104.7542, 118.2489) (104.4524, 118.099) (104.1518, 117.9475) (103.8525, 117.7944) (103.5544, 117.6397) (103.2576, 117.4832) (102.9622, 117.3252) (102.6681, 117.1654) (102.3753, 117.0039) (102.084, 116.8407) (101.794, 116.6758) (101.5053, 116.5091) (101.2182, 116.3408) (100.9325, 116.1707) (100.6483, 115.9987) (100.3659, 115.8247) (100.0853, 115.6487) (99.8064, 115.4706) (99.5293, 115.2905) (99.2539, 115.1085) (98.9801, 114.9246) (98.7078, 114.739) (98.4372, 114.5515) (98.1686, 114.3619) (97.9023, 114.1697) (97.6389, 113.9745) (97.3785, 113.7762) (97.1212, 113.5746) (96.8666, 113.3704) (96.614, 113.164) (96.3629, 112.956) (96.1132, 112.7467) (95.8657, 112.5352) (95.6223, 112.3199) (95.3854, 112.0982) (95.2033, 111.9138) (95.0718, 111.7706) (94.9865, 111.6729) (94.9444, 111.6235) knots -1 -1 -1 -1 -1 -1 -0.98571429 -0.97142857 -0.95714286 -0.94285714 -0.92857143 -0.91428571 -0.9 -0.88571429 -0.87142857 -0.85714286 -0.84285714 -0.82857143 -0.81428571 -0.8 -0.78571429 -0.77142857 -0.75714286 -0.74285714 -0.72857143 -0.71428571 -0.7 -0.68571429 -0.67142857 -0.65714286 -0.64285714 -0.62857143 -0.61428571 -0.6 -0.58571429 -0.57142857 -0.55714286 -0.54285714 -0.52857143 -0.51428571 -0.5 -0.48571429 -0.47142857 -0.45714286 -0.44285714 -0.42857143 -0.41428571 -0.4 -0.38571429 -0.37142857 -0.35714286 -0.34285714 -0.32857143 -0.31428571 -0.3 -0.28571429 -0.27142857 -0.25714286 -0.24285714 -0.22857143 -0.21428571 -0.2 -0.18571429 -0.17142857 -0.15714286 -0.14285714 -0.12857143 -0.11428571 -0.1 -0.08571429 -0.07142857 -0.05714286 -0.04285714 -0.02857143 -0.01428571 0 0 0 0 0 0
  line L31 (94.9444, 111.6235) -> (92.0135, 108.1802)
  arc A63 (89.7898, 107.9884) -> (92.0135, 108.1802) centre (90.8047, 109.2091) ccw
  arc A64 (89.7898, 107.9884) -> (81.2867, 114.513) centre (2.1352, 2.5578) ccw
  arc A65 (80.8964, 116.7107) -> (81.2867, 114.513) centre (82.2032, 115.8093) ccw
  line L32 (80.8964, 116.7107) -> (83.4638, 120.4328)